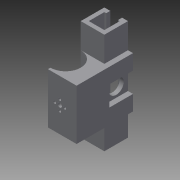
# Autodesk Inventor part: final_bracket
Saved by Autodesk Inventor 2015 (Build 190159000, 159)
## iProperties
Created: 2014-12-17
Part Number: final_bracket
Material: Generic
Document SubType Name: Modeling
Designer: Rene
Density: 1 g/cm^3
Appearance: Default
Author: Rene
Autodesk Inventor part; units mm, degrees
ref_plane "YZ Plane" through (0, 0, 0) normal (1, 0, 0) x (0, 1, 0)
ref_plane "XZ Plane" through (0, 0, 0) normal (0, 1, 0) x (-1, 0, 0)
ref_plane "XY Plane" through (0, 0, 0) normal (0, 0, 1) x (1, 0, 0)
sketch "Sketch1" plane through (0, 0, 0) normal (0, 1, 0) x (-1, 0, 0)
  line L0 (12.7, 12.7) -> (-12.7, 12.7)
  line L1 (-12.7, 12.7) -> (-12.7, -12.7)
  line L2 (-12.7, -12.7) -> (12.7, -12.7)
  line L3 (12.7, -12.7) -> (12.7, 12.7)
  point P0 (0, 0)
  dimension "d0" = 12.7
  dimension "d1" = 12.7
  dimension "d2" = 25.4
  dimension "d3" = 25.4
  constraints: 8 end point, 2 parallel, 1 horizontal, 1 perpendicular
  measures "d0" distance from line of point (0, 0) L3
  measures "d1" distance from line of point (0, 0) L2
  measures "d2" distance of L2.end L0.start
  measures "d3" distance of L0.start L0.end
extrude "Extrusion1" add sketch "Sketch1" along normal blind 101.6
sketch "Sketch2" plane through (0, 101.6, 0) normal (0, 1, 0) x (1, 0, 0)
  line L0 (-9.779, -9.779) -> (9.779, -9.779)
  line L1 (9.779, -9.779) -> (9.779, 9.779)
  line L2 (9.779, 9.779) -> (-9.779, 9.779)
  line L3 (-9.779, 9.779) -> (-9.779, -9.779)
  line L4 (-12.7, 12.7) -> (-12.7, -12.7) projected
  line L5 (-12.7, -12.7) -> (12.7, -12.7) projected
  line L6 (12.7, -12.7) -> (12.7, 12.7) projected
  line L7 (12.7, 12.7) -> (-12.7, 12.7) projected
  point P0 (0, 0)
  dimension "d6" = 2.921
  dimension "d7" = 2.921
  dimension "d8" = 2.921
  dimension "d9" = 2.921
  constraints: 8 end point, 2 parallel, 1 horizontal, 1 perpendicular
  measures "d6" distance between parallel lines of L4 L3
  measures "d7" distance between parallel lines of L5 L0
  measures "d8" distance between parallel lines of L6 L1
  measures "d9" distance between parallel lines of L7 L2
extrude "Extrusion2" cut sketch "Sketch2" against normal blind 101.6 contours L3 L2 L1 L0
sketch "Sketch3" plane through (0, 101.6, 0) normal (0, 1, 0) x (1, 0, 0)
  line L0 (-9.779, 9.779) -> (9.779, 9.779) projected
  line L1 (12.7, 12.7) -> (-12.7, 12.7) projected
  line L2 (-7.4168, 9.779) -> (7.4168, 9.779)
  line L3 (7.4168, 9.779) -> (7.4168, 12.7)
  line L4 (7.4168, 12.7) -> (-7.4168, 12.7)
  line L5 (-7.4168, 12.7) -> (-7.4168, 9.779)
  line L6 (-12.7, 12.7) -> (-12.7, -12.7) projected
  line L7 (12.7, -12.7) -> (12.7, 12.7) projected
  point P0 (0, 0)
  dimension "d12" = 5.2832
  dimension "d13" = 5.2832
  constraints: 8 end point, 2 parallel, 2 point on line, 1 horizontal, 1 perpendicular
  measures "d12" distance between parallel lines of L6 L5
  measures "d13" distance between parallel lines of L7 L3
extrude "Extrusion3" cut sketch "Sketch3" against normal blind 101.6
sketch "Sketch5" plane through (-12.7, 0, -12.7) normal (-1, 0, 0) x (0, 0, 1)
  line L0 (2.921, 40.005) -> (22.479, 40.005)
  line L1 (22.479, 40.005) -> (22.479, 81.3308)
  line L2 (22.479, 81.3308) -> (2.921, 81.3308)
  line L3 (2.921, 81.3308) -> (2.921, 40.005)
  line L4 (0, 0) -> (0, 101.6) projected
  line L5 (22.479, 101.6) -> (2.921, 101.6) projected
  point P0 (12.7, 0)
  dimension "d16" = 19.558
  dimension "d17" = 2.921
  dimension "d18" = 20.2692
  dimension "d19" = 41.3258
  constraints: 8 end point, 2 parallel, 1 horizontal, 1 perpendicular
  measures "d16" distance between parallel lines of L1 L3
  measures "d17" distance between parallel lines of L4 L3
  measures "d18" distance between parallel lines of L5 L2
  measures "d19" distance of L2.end L0.start
extrude "Extrusion4" cut sketch "Sketch5" against normal blind 5.08
sketch "Sketch6" plane through (-12.7, 0, -12.7) normal (-1, 0, 0) x (0, 0, 1)
  circle A0 centre (17.8308, 36.83) radius 3.175
  line L0 (25.4, 0) -> (25.4, 101.6) projected
  circle A1 centre (7.5692, 36.83) radius 3.175
  circle A2 centre (17.8308, 84.5058) radius 3.175
  circle A3 centre (7.5692, 84.5058) radius 3.175
  line L1 (0, 101.6) -> (25.4, 101.6) projected
  point P0 (12.7, 0)
  dimension "d22" = 7.5692
  dimension "d23" = 10.2616
  dimension "d24" = 6.35
  dimension "d25" = 6.35
  dimension "d26" = 6.35
  dimension "d27" = 6.35
  dimension "d28" = 17.0942
  dimension "d29" = 17.0942
  dimension "d30" = 10.2616
  dimension "d31" = 7.5692
  dimension "d32" = 47.6758
  dimension "d33" = 47.6758
  constraints: 4 centre point
  measures "d22" distance from line of L0 A0.centre
  measures "d23" distance of A1.centre A0.centre
  measures "d24" diameter of A1
  measures "d25" diameter of A0
  measures "d26" diameter of A2
  measures "d27" diameter of A3
  measures "d28" distance from line of L1 A2.centre
  measures "d29" distance from line of L1 A3.centre
  measures "d30" distance of A3.centre A2.centre
  measures "d31" distance from line of L0 A2.centre
  measures "d32" distance of A1.centre A3.centre
  measures "d33" distance of A2.centre A0.centre
extrude "Extrusion5" add sketch "Sketch6" along normal blind 3.3528
hole "Hole1" at (-16.0528, 84.5058, 5.1308) direction (1, 0, 0) diameter 1.651 depth 12.7 tip angle 118
hole "Hole2" at (-16.0528, 84.5058, -5.1308) direction (1, 0, 0) diameter 1.651 depth 12.7 tip angle 118
hole "Hole3" at (-16.0528, 36.83, 5.1308) direction (1, 0, 0) diameter 1.651 depth 12.7 tip angle 118
hole "Hole4" at (-16.0528, 36.83, -5.1308) direction (1, 0, 0) diameter 1.651 depth 12.7 tip angle 118
sketch "Sketch11" plane through (-12.7, 0, 12.7) normal (0, 0, 1) x (1, 0, 0)
  line L0 (5.08, 31.75) -> (17.78, 31.75)
  line L1 (17.78, 31.75) -> (17.78, 69.85)
  line L2 (17.78, 69.85) -> (5.08, 69.85)
  line L3 (5.08, 69.85) -> (5.08, 31.75)
  line L4 (0, 0) -> (25.4, 0) projected
  line L5 (0, 101.6) -> (25.4, 101.6) projected
  line L6 (0, 0) -> (0, 101.6) projected
  point P0 (12.7, 0)
  dimension "d82" = 31.75
  dimension "d83" = 31.75
  dimension "d84" = 5.08
  dimension "d85" = 12.7
  constraints: 8 end point, 2 parallel, 1 horizontal, 1 perpendicular
  measures "d82" distance between parallel lines of L4 L0
  measures "d83" distance between parallel lines of L5 L2
  measures "d84" distance between parallel lines of L6 L3
  measures "d85" distance of L0.start L0.end
extrude "Extrusion6" cut sketch "Sketch11" against normal blind 10.16
sketch "Sketch12" plane through (0, 0, 0) normal (0, -1, 0) x (1, 0, 0)
  line L0 (-7.4168, -9.779) -> (-7.4168, -14.859)
  line L1 (-7.4168, -14.859) -> (-14.859, -14.859)
  line L2 (-14.859, -14.859) -> (-14.859, 14.859)
  line L3 (-12.7, -12.7) -> (-12.7, 12.7) projected
  line L4 (-7.4168, -12.7) -> (-12.7, -12.7) projected
  line L5 (7.4168, -9.779) -> (7.4168, -14.859)
  line L6 (7.4168, -9.779) -> (7.4168, -12.7) projected
  line L7 (7.4168, -14.859) -> (14.859, -14.859)
  line L8 (14.859, -14.859) -> (14.859, 14.859)
  line L9 (12.7, -12.7) -> (7.4168, -12.7) projected
  line L10 (12.7, 12.7) -> (12.7, -12.7) projected
  line L11 (14.859, 14.859) -> (-14.859, 14.859)
  line L12 (5.08, 12.7) -> (-7.62, 12.7) projected
  line L13 (-7.4168, -12.7) -> (-7.4168, -9.779)
  line L14 (-7.4168, -12.7) -> (-7.4168, -9.779) projected
  line L15 (-9.779, -9.779) -> (-9.779, 9.779)
  line L16 (-9.779, 9.779) -> (9.779, 9.779) projected
  line L17 (-9.779, 9.779) -> (9.779, 9.779)
  line L18 (9.779, 9.779) -> (-9.779, 9.779) projected
  line L19 (9.779, 9.779) -> (9.779, -9.779)
  line L20 (9.779, -9.779) -> (7.4168, -9.779)
  line L21 (7.4168, -9.779) -> (9.779, -9.779) projected
  line L22 (-7.4168, -9.779) -> (-9.779, -9.779)
  point P0 (0, 0)
  dimension "d88" = 5.08
  dimension "d89" = 2.159
  dimension "d90" = 2.159
  dimension "d92" = 2.159
  dimension "d94" = 2.159
  dimension "d95" = 2.159
  constraints: 26 end point, 5 perpendicular, 4 collinear, 3 horizontal, 1 vertical
  measures "d88" distance of L0.start L0.end
  measures "d89" distance between parallel lines of L3 L2
  measures "d90" distance between parallel lines of L1 L4
  measures "d92" distance between parallel lines of L7 L9
  measures "d94" distance between parallel lines of L8 L10
  measures "d95" distance between parallel lines of L12 L11
extrude "Extrusion7" add sketch "Sketch12" against normal blind 101.6
hole "Hole5" at (-16.0528, 84.5058, 5.1308) direction (1, 0, 0) diameter 1.651 depth 12.7 tip angle 118
hole "Hole6" at (-16.0528, 84.5058, -5.1308) direction (1, 0, 0) diameter 1.651 depth 12.7 tip angle 118
hole "Hole7" at (-16.0528, 36.83, 5.1308) direction (1, 0, 0) diameter 1.651 depth 12.7 tip angle 118
hole "Hole8" at (-16.0528, 36.83, -5.1308) direction (1, 0, 0) diameter 1.651 depth 12.7 tip angle 118
sketch "Sketch13" plane through (-14.859, 0, -14.859) normal (-1, 0, 0) x (0, 0, 1)
  line L0 (5.08, 40.005) -> (24.638, 40.005)
  line L1 (24.638, 40.005) -> (24.638, 81.3308)
  line L2 (24.638, 81.3308) -> (5.08, 81.3308)
  line L3 (5.08, 81.3308) -> (5.08, 40.005)
  line L4 (0, 0) -> (0, 101.6) projected
  line L5 (29.718, 0) -> (29.718, 101.6) projected
  line L6 (0, 101.6) -> (29.718, 101.6) projected
  point P0 (14.859, 0)
  dimension "d136" = 41.3258
  dimension "d137" = 20.2692
  dimension "d139" = 19.558
  dimension "d140" = 29.718
  dimension "d141" = 5.08
  dimension "d142" = 5.08
  constraints: 8 end point, 2 parallel, 1 horizontal, 1 perpendicular
  measures "d136" distance between parallel lines of L2 L0
  measures "d137" distance between parallel lines of L6 L2
  measures "d139" distance between parallel lines of L1 L3
  measures "d140" distance between parallel lines of L5 L4
  measures "d141" distance between parallel lines of L4 L3
  measures "d142" distance between parallel lines of L5 L1
extrude "Extrusion8" cut sketch "Sketch13" against normal blind 10.16
sketch "Sketch15" plane through (-14.859, 0, 14.859) normal (0, 0, 1) x (1, 0, 0)
  line L0 (5.08, 31.75) -> (24.13, 31.75)
  line L1 (24.13, 31.75) -> (24.13, 69.85)
  line L2 (24.13, 69.85) -> (5.08, 69.85)
  line L3 (5.08, 69.85) -> (5.08, 31.75)
  line L4 (0, 101.6) -> (29.718, 101.6) projected
  line L5 (0, 0) -> (0, 101.6) projected
  line L6 (29.718, 0) -> (29.718, 101.6) projected
  point P0 (14.859, 0)
  dimension "d145" = 38.1
  dimension "d146" = 31.75
  dimension "d147" = 19.05
  dimension "d148" = 5.08
  constraints: 8 end point, 2 parallel, 1 horizontal, 1 perpendicular
  measures "d145" distance of L2.end L0.start
  measures "d146" distance between parallel lines of L4 L2
  measures "d147" distance of L0.start L0.end
  measures "d148" distance between parallel lines of L5 L3
extrude "Extrusion9" cut sketch "Sketch15" against normal blind 10.16
chamfer "Chamfer1" distance 5.08 angle 45 2 edges at (-0.254, 69.85, 9.779) (-0.254, 31.75, 9.779)
sketch "Sketch17" plane through (0, 101.6, 0) normal (0, 1, 0) x (1, 0, 0)
  line L0 (-7.4168, 9.779) -> (-7.4168, 14.859)
  line L1 (-7.4168, 14.859) -> (-14.859, 14.859)
  line L2 (-14.859, 14.859) -> (-14.859, -14.859)
  line L3 (-14.859, -14.859) -> (14.859, -14.859)
  line L4 (14.859, -14.859) -> (14.859, 14.859)
  line L5 (14.859, 14.859) -> (14.859, -14.859) projected
  line L6 (14.859, 14.859) -> (7.4168, 14.859)
  line L7 (7.4168, 14.859) -> (7.4168, 9.779)
  line L8 (7.4168, 9.779) -> (7.4168, 14.859) projected
  line L9 (7.4168, 9.779) -> (9.779, 9.779)
  line L10 (9.779, 9.779) -> (9.779, -9.779)
  line L11 (9.779, -9.779) -> (-9.779, -9.779)
  line L12 (-9.779, -9.779) -> (9.779, -9.779) projected
  line L13 (-9.779, -9.779) -> (-9.779, 9.779)
  line L14 (-9.779, -9.779) -> (-9.779, 9.779) projected
  line L15 (-9.779, 9.779) -> (-7.4168, 9.779)
  line L16 (-7.4168, 9.779) -> (-9.779, 9.779) projected
  line L17 (-7.4168, 9.779) -> (-7.4168, 14.859)
  point P0 (0, 0)
  constraints: 26 end point, 7 perpendicular, 5 collinear, 1 vertical
extrude "Extrusion10" add sketch "Sketch17" along normal blind 12.7
sketch "Sketch18" plane through (0, 0, 0) normal (0, -1, 0) x (1, 0, 0)
  line L0 (-7.4168, -9.779) -> (-7.4168, -14.859)
  line L1 (-7.4168, -14.859) -> (-7.4168, -9.779) projected
  line L2 (-7.4168, -14.859) -> (-14.859, -14.859)
  line L3 (-14.859, -14.859) -> (-7.4168, -14.859) projected
  line L4 (-14.859, -14.859) -> (-14.859, 14.859)
  line L5 (-14.859, 14.859) -> (14.859, 14.859)
  line L6 (14.859, 14.859) -> (-14.859, 14.859) projected
  line L7 (14.859, 14.859) -> (14.859, -14.859)
  line L8 (14.859, -14.859) -> (7.4168, -14.859)
  line L9 (7.4168, -14.859) -> (7.4168, -9.779)
  line L10 (7.4168, -9.779) -> (7.4168, -14.859) projected
  line L11 (7.4168, -9.779) -> (9.779, -9.779)
  line L12 (9.779, -9.779) -> (9.779, 9.779)
  line L13 (9.779, 9.779) -> (9.779, -9.779) projected
  line L14 (9.779, 9.779) -> (-9.779, 9.779)
  line L15 (-9.779, 9.779) -> (-9.779, -9.779)
  line L16 (-9.779, -9.779) -> (-9.779, 9.779) projected
  line L17 (-9.779, -9.779) -> (-7.4168, -9.779)
  line L18 (-7.4168, -9.779) -> (-9.779, -9.779) projected
  line L19 (-7.4168, -14.859) -> (-14.859, -14.859)
  point P0 (0, 0)
  constraints: 26 end point, 8 collinear, 5 perpendicular
extrude "Extrusion11" add sketch "Sketch18" along normal blind 12.7
sketch "Sketch20" plane through (14.859, 114.3, 14.859) normal (1, 0, 0) x (0, 0, -1)
  circle A0 centre (14.859, -63.5) radius 9.525
  line L0 (29.718, -127) -> (0, -127) projected
  line L1 (0, 0) -> (0, -127) projected
  line L2 (29.718, 0) -> (29.718, -127) projected
  point P0 (14.859, -114.3)
  dimension "d160" = 63.5
  dimension "d161" = 19.05
  dimension "d162" = 14.859
  dimension "d163" = 29.718
  constraints: 1 centre point
  measures "d160" distance from line of L0 A0.centre
  measures "d161" diameter of A0
  measures "d162" distance from line of L1 A0.centre
  measures "d163" distance between parallel lines of L2 L1
extrude "Extrusion12" cut sketch "Sketch20" against normal blind 12.7
sketch "Sketch21" plane through (14.859, 114.3, 14.859) normal (1, 0, 0) x (0, 0, -1)
  line L0 (0, 0) -> (0, -127) projected
  line L1 (29.718, 0) -> (29.718, -127) projected
  line L2 (0, -95.25) -> (29.718, -95.25)
  line L3 (29.718, -95.25) -> (29.718, -76.2)
  line L4 (29.718, -76.2) -> (0, -76.2)
  line L5 (0, -76.2) -> (0, -95.25)
  circle A0 centre (14.859, -63.5) radius 9.525 projected
  line L6 (0, -50.8) -> (29.718, -50.8)
  line L7 (29.718, -50.8) -> (29.718, -31.75)
  line L8 (29.718, -31.75) -> (0, -31.75)
  line L9 (0, -31.75) -> (0, -50.8)
  point P0 (14.859, -114.3)
  dimension "d166" = 12.7
  dimension "d167" = 19.05
  dimension "d168" = 12.7
  dimension "d169" = 19.05
  constraints: 16 end point, 4 parallel, 4 point on line, 2 horizontal, 2 perpendicular
  measures "d166" distance from line of A0.centre L4
  measures "d167" distance between parallel lines of L4 L2
  measures "d168" distance from line of A0.centre L6
  measures "d169" distance between parallel lines of L6 L8
extrude "Extrusion13" add sketch "Sketch21" along normal blind 6.35 contours L8 L1 L6 L0 | L4 L1 L2 L0
sketch "Sketch22" plane through (-14.859, 114.3, 14.859) normal (0, 0, 1) x (1, 0, 0)
  line L0 (36.068, -95.25) -> (29.718, -95.25)
  line L1 (29.718, -95.25) -> (29.718, -31.75)
  line L2 (29.718, -31.75) -> (36.068, -31.75)
  line L3 (36.068, -31.75) -> (36.068, -95.25)
  point P0 (14.859, -114.3)
  constraints: 8 end point, 2 parallel, 1 horizontal, 1 perpendicular
extrude "Extrusion14" add sketch "Sketch22" along normal blind 63.5
sketch "Sketch23" plane through (-14.859, 114.3, 78.359) normal (0, 0, 1) x (1, 0, 0)
  line L0 (29.718, -95.25) -> (29.718, -127) projected
  line L1 (0, 0) -> (0, -127) projected
  line L2 (0, 0) -> (29.718, 0) projected
  line L3 (29.718, -127) -> (0, -127) projected
  circle A0 centre (14.859, -63.5) radius 2.7305
  circle A1 centre (14.859, -57.15) radius 1.651
  circle A2 centre (8.509, -63.5) radius 1.651
  circle A3 centre (14.859, -69.85) radius 1.651
  circle A4 centre (21.209, -63.5) radius 1.651
  line L4 (36.068, -95.25) -> (0, -95.25)
  line L5 (0, -95.25) -> (0, -31.75)
  line L6 (0, -31.75) -> (36.068, -31.75)
  line L7 (36.068, -31.75) -> (36.068, -95.25)
  point P0 (14.859, -114.3)
  dimension "d174" = 29.718
  dimension "d175" = 127
  dimension "d176" = 63.5
  dimension "d177" = 14.859
  dimension "d178" = 5.461
  dimension "d179" = 6.35
  dimension "d180" = 3.302
  dimension "d181" = 0
  dimension "d182" = 6.35
  dimension "d183" = 3.302
  dimension "d184" = 6.35
  dimension "d185" = 0
  dimension "d186" = 3.302
  dimension "d187" = 6.35
  dimension "d188" = 0
  dimension "d189" = 3.302
  dimension "d190" = 63.5
  dimension "d191" = 0
  constraints: 8 end point, 5 centre point, 2 parallel, 1 horizontal, 1 perpendicular
  measures "d174" distance between parallel lines of L0 L1
  measures "d175" distance between parallel lines of L2 L3
  measures "d176" distance from line of L3 A0.centre
  measures "d177" distance from line of L1 A0.centre
  measures "d178" diameter of A0
  measures "d179" distance of A1.centre A0.centre
  measures "d180" diameter of A1
  measures "d181" vertical distance of A0.centre A2.centre
  measures "d182" distance of A0.centre A2.centre
  measures "d183" diameter of A2
  measures "d184" distance of A0.centre A3.centre
  measures "d185" horizontal distance of A0.centre A3.centre
  measures "d186" diameter of A3
  measures "d187" distance of A4.centre A0.centre
  measures "d188" vertical distance of A0.centre A4.centre
  measures "d189" diameter of A4
  measures "d190" distance between parallel lines of L6 L4
  measures "d191" distance between parallel lines of L1 L5
extrude "Extrusion15" add sketch "Sketch23" against normal blind 63.5 contours L4 L1 L6 L7
sketch "Sketch24" plane through (-14.859, 114.3, -14.859) normal (-1, 0, 0) x (0, 0, 1)
  line L0 (29.718, -34.925) -> (67.818, -34.925)
  line L1 (67.818, -34.925) -> (67.818, -92.075)
  line L2 (67.818, -92.075) -> (29.718, -92.075)
  line L3 (29.718, -92.075) -> (29.718, -34.925)
  line L4 (29.718, -95.25) -> (29.718, -127) projected
  line L5 (93.218, -95.25) -> (29.718, -95.25) projected
  line L6 (93.218, -31.75) -> (29.718, -31.75) projected
  point P0 (14.859, -114.3)
  dimension "d194" = 38.1
  dimension "d195" = 0
  dimension "d196" = 3.175
  dimension "d197" = 3.175
  constraints: 8 end point, 2 parallel, 1 horizontal, 1 perpendicular
  measures "d194" distance of L1.end L2.end
  measures "d195" distance between parallel lines of L4 L3
  measures "d196" distance between parallel lines of L5 L2
  measures "d197" distance between parallel lines of L6 L0
extrude "Extrusion16" cut sketch "Sketch24" against normal blind 30.48
sketch "Sketch26" plane through (-14.859, 114.3, -14.859) normal (-1, 0, 0) x (0, 0, 1)
  line L0 (93.218, -95.25) -> (29.718, -95.25) projected
  line L1 (70.993, -95.25) -> (70.993, -31.75)
  line L2 (93.218, -31.75) -> (29.718, -31.75) projected
  line L3 (67.818, -34.925) -> (67.818, -92.075) projected
  line L4 (70.993, -95.25) -> (93.218, -95.25)
  line L5 (93.218, -31.75) -> (70.993, -31.75)
  line L6 (93.218, -95.25) -> (70.993, -95.25)
  line L7 (70.993, -95.25) -> (70.993, -31.75)
  line L8 (70.993, -31.75) -> (93.218, -31.75)
  line L9 (93.218, -31.75) -> (93.218, -95.25)
  point P0 (14.859, -114.3)
  dimension "d200" = 3.175
  constraints: 14 end point, 2 collinear, 2 parallel, 2 point on line, 1 horizontal, 1 perpendicular, 1 vertical
  measures "d200" distance between parallel lines of L3 L1
extrude "Extrusion17" cut sketch "Sketch26" against normal blind 50.8
sketch "Sketch27" plane through (14.859, 82.55, 14.859) normal (0, 1, 0) x (1, 0, 0)
  line L0 (-29.718, 0) -> (-29.718, -38.1) projected
  circle A0 centre (-29.718, -19.05) radius 19.05
  line L1 (-29.718, 0) -> (0, 0) projected
  line L2 (-29.718, -38.1) -> (0.762, -38.1) projected
  point P0 (-14.859, 14.859)
  dimension "d203" = 38.1
  dimension "d204" = 19.05
  dimension "d205" = 38.1
  constraints: 1 centre point, 1 midpoint
  measures "d203" distance between parallel lines of L1 L2
  measures "d204" distance from line of L2 A0.centre
  measures "d205" diameter of A0
extrude "Extrusion18" cut sketch "Sketch27" against normal blind 101.6
sketch "Sketch30" plane through (-9.779, 40.005, 9.779) normal (0, 0, -1) x (-1, 0, 0)
  line L0 (-19.05, 34.925) -> (-14.7718, 34.925)
  line L1 (-14.7718, 34.925) -> (-14.7718, -14.5025)
  line L2 (-14.7718, -14.5025) -> (-19.05, -14.5025)
  line L3 (-19.05, -14.5025) -> (-19.05, 34.925)
  point P0 (-9.779, -40.005)
  constraints: 8 end point, 2 parallel, 1 horizontal, 1 perpendicular
extrude "Extrusion19" add sketch "Sketch30" against normal blind 5.08
body "Solid1"
